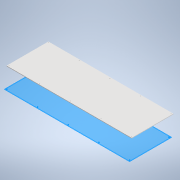
# Autodesk Inventor part: base
Saved by Autodesk Inventor 2021 (Build 250183000, 183)
## iProperties
Created: 2022-01-22
Part Number: base
Material: Generic
Document SubType Name: Modeling
Designer: avan411
Density: 1 g/cm^3
Appearance: Default
Author: avan411
Autodesk Inventor part; units mm, degrees
ref_plane "YZ Plane" through (0, 0, 0) normal (1, 0, 0) x (0, 1, 0)
ref_plane "XZ Plane" through (0, 0, 0) normal (0, 1, 0) x (-1, 0, 0)
ref_plane "XY Plane" through (0, 0, 0) normal (0, 0, 1) x (1, 0, 0)
sketch "Sketch1" plane through (0, 0, 0) normal (0, 1, 0) x (-1, 0, 0)
  line L0 (-125.004, -326.6241) -> (924.996, -326.6241) projected
  line L1 (924.996, -326.6241) -> (924.996, 23.3759) projected
  line L2 (924.996, 23.3759) -> (-125.004, 23.3759) projected
  line L3 (-125.004, 23.3759) -> (-125.004, -326.6241) projected
  line L4 (924.996, 23.3759) -> (-125.004, 23.3759) projected
  line L5 (-125.004, 23.3759) -> (-125.004, -326.6241) projected
  line L6 (-125.004, -326.6241) -> (924.996, -326.6241) projected
  line L7 (924.996, -326.6241) -> (924.996, 23.3759) projected
  line L8 (-100.004, -1.6241) -> (899.996, -1.6241) projected
  line L9 (899.996, -1.6241) -> (899.996, -301.6241) projected
  line L10 (899.996, -301.6241) -> (-100.004, -301.6241) projected
  line L11 (-100.004, -301.6241) -> (-100.004, -1.6241) projected
  circle A0 centre (399.996, -316.6241) radius 3 projected
  circle A1 centre (914.996, -316.6241) radius 3 projected
  circle A2 centre (-115.004, -316.6241) radius 3 projected
  circle A3 centre (142.496, -316.6241) radius 3 projected
  circle A4 centre (399.996, 13.3759) radius 3 projected
  circle A5 centre (142.496, 13.3759) radius 3 projected
  circle A6 centre (-115.004, 13.3759) radius 3 projected
  circle A7 centre (657.496, 13.3759) radius 3 projected
  circle A8 centre (914.996, 13.3759) radius 3 projected
  circle A9 centre (657.496, -316.6241) radius 3 projected
  point P0 (0, 0)
extrude "Extrusion1" add sketch "Sketch1" along normal blind 5 contours L3 L2 L1 L0 | L8 L9 L10 L11
body "Solid1"
